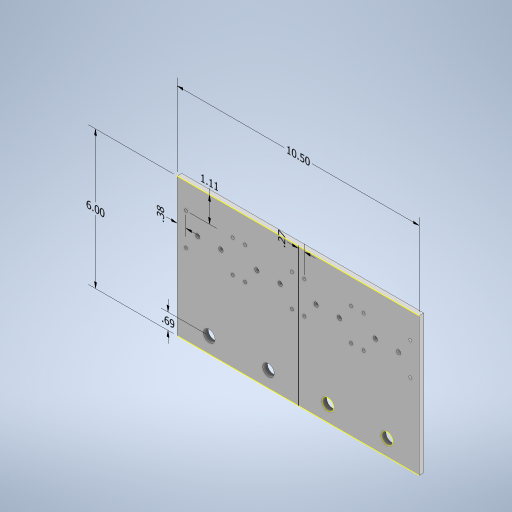
# Autodesk Inventor part: Back wall
Saved by Autodesk Inventor 2024.3 (Build 283343010, 343A)
## iProperties
Created: 2025-04-08
Part Number: Back wall
Material: Generic
Document SubType Name: Modeling
Designer: Vincent Larson
Density: 1 g/cm^3
Appearance: Default
Author: Vincent Larson
Autodesk Inventor part; units mm, degrees
ref_plane "YZ Plane" through (0, 0, 0) normal (1, 0, 0) x (0, 1, 0)
ref_plane "XZ Plane" through (0, 0, 0) normal (0, 1, 0) x (-1, 0, 0)
ref_plane "XY Plane" through (0, 0, 0) normal (0, 0, 1) x (1, 0, 0)
sketch "Sketch3" plane through (0, 0, 0) normal (0, 0, 1) x (1, 0, 0)
  line L0 (0, 0) -> (266.7, 0)
  line L1 (266.7, 0) -> (266.7, -152.4)
  line L2 (266.7, -152.4) -> (0, -152.4)
  line L3 (0, -152.4) -> (0, 0)
  dimension "d8" = 266.7
  dimension "d9" = 152.4
  constraints: 8 end point, 2 parallel, 1 horizontal, 1 perpendicular
  measures "d8" distance of L1.end L2.end
  measures "d9" distance of L0.end L1.end
extrude "Extrusion3" add sketch "Sketch3" along normal blind 5.08
sketch "Sketch4" plane through (0, 0, 5.08) normal (0, 0, 1) x (1, 0, 0)
  line L0 (0, -152.4) -> (266.7, -152.4) projected
  line L1 (266.7, 0) -> (0, 0) projected
  line L2 (133.35, 0) -> (133.35, -152.4)
  line L3 (266.7, -152.4) -> (266.7, 0) projected
  circle A0 centre (126.492, -28.2016) radius 1.651
  circle A1 centre (140.208, -28.2016) radius 1.651
  circle A2 centre (191.77, -28.2016) radius 1.651
  circle A3 centre (74.93, -28.2016) radius 1.651
  circle A4 centre (205.486, -28.2016) radius 1.651
  circle A5 centre (61.214, -28.2016) radius 1.651
  circle A6 centre (257.048, -28.2016) radius 1.651
  circle A7 centre (9.652, -28.2016) radius 1.651
  circle A8 centre (140.208, -63.7616) radius 1.651
  circle A9 centre (126.492, -63.7616) radius 1.651
  circle A10 centre (191.77, -63.7616) radius 1.651
  circle A11 centre (74.93, -63.7616) radius 1.651
  circle A12 centre (205.486, -63.7616) radius 1.651
  circle A13 centre (61.214, -63.7616) radius 1.651
  circle A14 centre (257.048, -63.7616) radius 1.651
  circle A15 centre (9.652, -63.7616) radius 1.651
  circle A16 centre (153.162, -45.9816) radius 2.413
  circle A17 centre (113.538, -45.9816) radius 2.413
  circle A18 centre (178.816, -45.9816) radius 2.413
  circle A19 centre (87.884, -45.9816) radius 2.413
  circle A20 centre (218.44, -45.9816) radius 2.413
  circle A21 centre (48.26, -45.9816) radius 2.413
  circle A22 centre (244.094, -45.9816) radius 2.413
  circle A23 centre (22.606, -45.9816) radius 2.413
  constraints: 24 centre point, 11 symmetric about line, 2 end point, 2 midpoint, 11 other
extrude "Extrusion5" cut sketch "Sketch4" against normal blind 25.4 contours A0 | A1 | A2 | A3 | A4 | A5 | A6 | A7 | A8 | A9 | A10 | A11 | A12 | A13 | A14 | A15 | A16 | A17 | A18 | A19 | A20 | A21 | A22 | A23
sketch "Sketch6" plane through (0, 0, 5.08) normal (0, 0, 1) x (1, 0, 0)
  circle A0 centre (22.606, -45.9816) radius 2.413 projected
  circle A1 centre (48.26, -45.9816) radius 2.413 projected
  circle A2 centre (87.884, -45.9816) radius 2.413 projected
  circle A3 centre (113.538, -45.9816) radius 2.413 projected
  line L0 (266.7, 0) -> (0, 0) projected
  line L1 (0, 0) -> (266.7, 0)
  line L2 (133.35, 0) -> (133.35, -152.4)
  line L3 (0, -152.4) -> (266.7, -152.4) projected
  circle A4 centre (35.433, -134.8816) radius 6.35
  circle A5 centre (100.711, -134.8816) radius 6.35
  circle A6 centre (231.267, -134.8816) radius 6.35
  circle A7 centre (165.989, -134.8816) radius 6.35
  dimension "d99" = 12.7
  dimension "d100" = 12.7
  constraints: 4 centre point, 4 end point, 2 midpoint, 2 symmetric about line, 1 collinear, 2 other
  measures "d99" diameter of A4
  measures "d100" diameter of A5
extrude "Extrusion6" cut sketch "Sketch6" against normal blind 25.4 contours A4 | A5 | A6 | A7
sketch "Sketch7" plane through (0, 0, 5.08) normal (0, 0, 1) x (1, 0, 0)
  point P0 (0, 0)
sketch "Sketch8" plane through (0, 0, 5.08) normal (0, 0, 1) x (1, 0, 0)
  line L0 (266.7, 0) -> (0, 0) projected
  line L1 (0, -152.4) -> (266.7, -152.4) projected
  circle A0 centre (165.989, -134.8816) radius 6.35 projected
  circle A1 centre (231.267, -134.8816) radius 6.35 projected
sketch "Sketch9" plane through (0, 0, 5.08) normal (0, 0, 1) x (1, 0, 0)
  line L0 (266.7, 0) -> (0, 0) projected
  line L1 (133.35, 0) -> (133.35, -152.4)
  line L2 (0, -152.4) -> (266.7, -152.4) projected
  constraints: 2 end point, 2 midpoint
body "Solid2"
